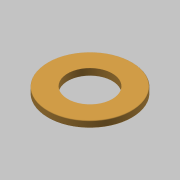
# Autodesk Inventor part: InputJack_partition1
Saved by Autodesk Inventor 2015 SP1 (Build 190203100, 203)
## iProperties
Created: 2015-06-13
Part Number: InputJack_partition1
Material: Generic
Document SubType Name: Modeling
Designer: Peter Mulkers
Density: 1 g/cm^3
Appearance: Orange
Author: Peter Mulkers
Autodesk Inventor part; units mm, degrees
ref_plane "YZ Plane" through (0, 0, 0) normal (1, 0, 0) x (0, 1, 0)
ref_plane "XZ Plane" through (0, 0, 0) normal (0, 1, 0) x (-1, 0, 0)
ref_plane "XY Plane" through (0, 0, 0) normal (0, 0, 1) x (1, 0, 0)
sketch "Sketch1" plane through (0, 0, 0) normal (0, 0, 1) x (1, 0, 0)
  circle A0 centre (0, 0) radius 9
  circle A1 centre (0, 0) radius 4.7625
  dimension "d0" = 18
  dimension "d1" = 9.525
  constraints: 2 centre point, 2 coincident
  measures "d0" diameter of A0
  measures "d1" diameter of A1
extrude "Extrusion1" add sketch "Sketch1" along normal blind 1.4
fillet "Fillet1" radius 0.15 2 edges at (-9, 0, 0) (-9, 0, 1.4)
body "Solid1"
